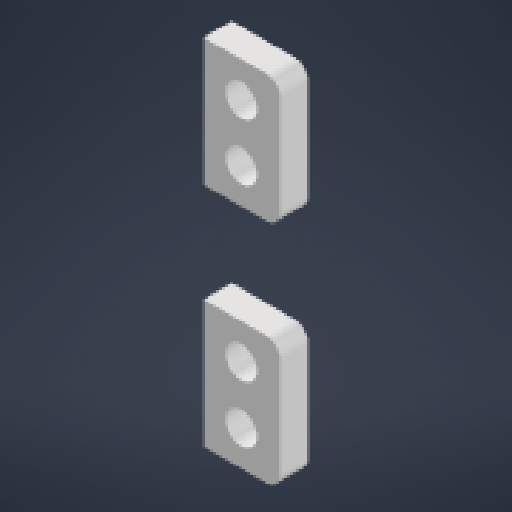
# Autodesk Inventor part: Adapter
Saved by Autodesk Inventor 2023.4 (Build 274418000, 418)
## iProperties
Created: 2025-10-16
Part Number: Adapter
Material: Generic
Document SubType Name: Modeling
Designer: Malthe Sennels
Density: 1 g/cm^3
Appearance: Default
Author: Malthe Sennels
Autodesk Inventor part; units mm, degrees
ref_plane "YZ Plane" through (0, 0, 0) normal (1, 0, 0) x (0, 1, 0)
ref_plane "XZ Plane" through (0, 0, 0) normal (0, 1, 0) x (-1, 0, 0)
ref_plane "XY Plane" through (0, 0, 0) normal (0, 0, 1) x (1, 0, 0)
sketch "Sketch1" plane through (0, 0, 0) normal (0, 0, 1) x (1, 0, 0)
  arc A0 (5.5, 7) -> (3.5, 9) centre (3.5, 7) ccw projected
  line L0 (3.5, 9) -> (-5.5, 9) projected
  line L1 (-5.5, -9) -> (-5.5, 9) projected
  line L2 (-5.5, -9) -> (3.5, -9) projected
  arc A1 (3.5, -9) -> (5.5, -7) centre (3.5, -7) ccw projected
  line L3 (5.5, -7) -> (5.5, 7) projected
  circle A2 centre (0, 4) radius 2.25 projected
  circle A3 centre (0, -4) radius 2.25 projected
  arc A4 (5.5, 39) -> (3.5, 41) centre (3.5, 39) ccw projected
  line L4 (3.5, 41) -> (-5.5, 41) projected
  line L5 (-5.5, 23) -> (-5.5, 41) projected
  line L6 (-5.5, 23) -> (3.5, 23) projected
  arc A5 (3.5, 23) -> (5.5, 25) centre (3.5, 25) ccw projected
  line L7 (5.5, 25) -> (5.5, 39) projected
  circle A6 centre (0, 36) radius 2.25 projected
  circle A7 centre (0, 28) radius 2.25 projected
  line L8 (-5.3, -9) -> (-5.3, 9)
  line L9 (-5.3, 23) -> (-5.3, 41)
  circle A8 centre (0, -4) radius 1.75
  circle A9 centre (0, 4) radius 1.75
  circle A10 centre (0, 28) radius 1.75
  circle A11 centre (0, 36) radius 1.75
  point P0 (0, 0)
  dimension "d0" = 0.2
  dimension "d1" = 0.2
  dimension "d4" = 3.5
  dimension "d5" = 3.5
  dimension "d6" = 3.5
  dimension "d7" = 3.5
  constraints: 4 centre point, 4 coincident, 4 end point, 4 point on line, 2 perpendicular
  measures "d0" distance between parallel lines of L1 L8
  measures "d1" distance between parallel lines of L5 L9
  measures "d4" diameter of A8
  measures "d5" diameter of A9
  measures "d6" diameter of A10
  measures "d7" diameter of A11
extrude "Extrusion1" add sketch "Sketch1" along normal blind 4 contours L3 A1 L2 L8 L0 A0 | A2 | A3 | L7 A5 L6 L9 L4 A4 | A6 | A7
body "Solid1"
